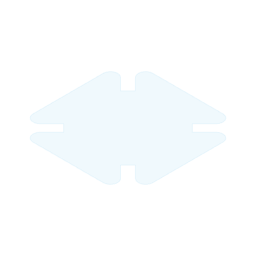
press-fit v4 (Autodesk Fusion 360 design; units mm, degrees)
Autodesk Fusion 360 part; units mm, degrees
sketch "Sketch1" plane through (0, 0, 0) normal (0, 0, 1) x (1, 0, 0)
sketch "Sketch2" plane through (0, 0, 0) normal (0, 0, 1) x (1, 0, 0)
  line L0 (-0.1061, 25.1061) -> (49.8939, 25.1061)
  line L1 (49.8939, 25.1061) -> (49.8939, -24.8939)
  line L2 (49.8939, -24.8939) -> (-0.1061, -24.8939)
  line L3 (-0.1061, -24.8939) -> (-0.1061, 25.1061)
  line L4 (9.8939, -14.8939) -> (9.8939, 15.1061)
  line L5 (9.8939, 15.1061) -> (39.8939, 15.1061)
  line L6 (39.8939, 15.1061) -> (39.8939, -14.8939)
  line L7 (39.8939, -14.8939) -> (9.8939, -14.8939)
  line L8 (-0.1061, -24.8939) -> (49.8939, 25.1061) construction
  line L9 (-0.1061, 25.1061) -> (49.8939, -24.8939) construction
  line L10 (-1.6263, -23.3737) -> (48.3737, 26.6264)
  line L11 (-1.6617, 23.5504) -> (48.3383, -26.4496)
  line L12 (1.4496, 26.6617) -> (51.4496, -23.3383)
  line L13 (1.4142, -26.4142) -> (51.4142, 23.5858)
  line L14 (12.9345, -14.8939) -> (9.8939, -11.8534)
  line L15 (36.7827, -14.8939) -> (39.8939, -11.7827)
  line L16 (9.8939, 11.9948) -> (13.0052, 15.1061)
  line L17 (36.8534, 15.1061) -> (39.8939, 12.0655)
  dimension "d10" = 50
  dimension "d11" = 50
  dimension "d12" = 10
  dimension "test" = 4.3
  dimension "test2" = 4.3
  constraint horizontal L0
  constraint vertical L1
  constraint horizontal L2
  constraint vertical L3
  constraint symmetric L9 L11.start L12.start
  constraint symmetric L9 L11.end L12.end
  constraint symmetric L8 L10.start L13.start
  constraint symmetric L8 L10.end L13.end
  constraint coincident L13 L14.start
  constraint coincident L7 L14.start
  constraint coincident L10 L14.end
  constraint coincident L4 L14.end
  constraint perpendicular L10 L14
  constraint coincident L7 L15.start
  constraint coincident L11 L15.start
  constraint coincident L6 L15.end
  constraint coincident L12 L15.end
  constraint perpendicular L12 L15
  constraint coincident L11 L16.start
  constraint coincident L4 L16.start
  constraint coincident L5 L16.end
  constraint coincident L12 L16.end
  constraint perpendicular L12 L16
  constraint coincident L5 L17.start
  constraint coincident L10 L17.start
  constraint coincident L6 L17.end
  constraint coincident L13 L17.end
  constraint perpendicular L13 L17
  measures "d10" distance of L0.start L0.end
  measures "d11" distance of L0.start L2.end
  measures "test" distance of L10 L13
extrude "Extrude3" add sketch "Sketch2" along normal blind 4.4 contours L0 L5 L10 L12 | L3 L4 L10 L11 | L5 L10 L12 | L10 L11 L12 L16 | L4 L10 L11 | L10 L12 L13 L17 | L10 L11 L12 L13 | L10 L11 L13 L14 | L1 L6 L12 L13 | L6 L12 L13 | L11 L12 L13 L15 | L2 L7 L11 L13 | L7 L11 L13 makes body 1
extrude "Extrude2" add sketch "Sketch2" along normal blind 4.4 separate body contours L0 L5 L10 L12 | L3 L4 L10 L11 | L5 L10 L12 | L10 L11 L12 L16 | L4 L10 L11 | L10 L12 L13 L17 | L10 L11 L12 L13 | L10 L11 L13 L14 | L1 L6 L12 L13 | L6 L12 L13 | L11 L12 L13 L15 | L2 L7 L11 L13 | L7 L11 L13 makes body 2
sketch "Sketch4" plane through (0, 0, 0) normal (0, 0, 1) x (1, 0, 0)
fillet "Fillet2" radius 3 8 edges at (49.8939, 22.0655, 2.2) (46.8534, 25.1061, 2.2) (3.0052, 25.1061, 2.2) (-0.1061, 21.9948, 2.2) (2.9345, -24.8939, 2.2) (46.7827, -24.8939, 2.2) (49.8939, -21.7827, 2.2) (-0.1061, -21.8534, 2.2) on bodies 2
sketch "Sketch5" plane through (0, 0, 4.4) normal (0, 0, 1) x (-1, 0, 0)
  arc A0 (0.1061, 14.6107) -> (-5.0153, 16.7321) centre (-2.8939, 14.6107) ccw
  line L0 (-5.0153, 16.7321) -> (-9.8939, 11.8534)
  line L1 (-9.8939, 11.8534) -> (-12.9345, 14.8939)
  line L2 (-12.9345, 14.8939) -> (-8.0558, 19.7726)
  arc A1 (-8.0558, 19.7726) -> (-10.1771, 24.8939) centre (-10.1771, 21.8939) ccw
  line L3 (-10.1771, 24.8939) -> (-39.54, 24.8939)
  arc A2 (-39.54, 24.8939) -> (-41.6613, 19.7726) centre (-39.54, 21.8939) ccw
  line L4 (-41.6613, 19.7726) -> (-36.7827, 14.8939)
  line L5 (-36.7827, 14.8939) -> (-39.8939, 11.7827)
  line L6 (-39.8939, 11.7827) -> (-44.7726, 16.6613)
  arc A3 (-44.7726, 16.6613) -> (-49.8939, 14.54) centre (-46.8939, 14.54) ccw
  line L7 (-49.8939, 14.54) -> (-49.8939, -14.8229)
  arc A4 (-49.8939, -14.8229) -> (-44.7726, -16.9442) centre (-46.8939, -14.8229) ccw
  line L8 (-44.7726, -16.9442) -> (-39.8939, -12.0655)
  line L9 (-39.8939, -12.0655) -> (-36.8534, -15.1061)
  line L10 (-36.8534, -15.1061) -> (-41.7321, -19.9847)
  arc A5 (-41.7321, -19.9847) -> (-39.6107, -25.1061) centre (-39.6107, -22.1061) ccw
  line L11 (-39.6107, -25.1061) -> (-10.2478, -25.1061)
  arc A6 (-10.2478, -25.1061) -> (-8.1265, -19.9847) centre (-10.2478, -22.1061) ccw
  line L12 (-8.1265, -19.9847) -> (-13.0052, -15.1061)
  line L13 (-13.0052, -15.1061) -> (-9.8939, -11.9948)
  line L14 (-9.8939, -11.9948) -> (-5.0153, -16.8735)
  arc A7 (-5.0153, -16.8735) -> (0.1061, -14.7522) centre (-2.8939, -14.7522) ccw
  line L15 (0.1061, -14.7522) -> (0.1061, 14.6107)
fillet "Fillet3" radius 3 8 edges at (46.7827, -24.8939, 2.2) (49.8939, -21.7827, 2.2) (2.9345, -24.8939, 2.2) (-0.1061, -21.8534, 2.2) (49.8939, 22.0655, 2.2) (46.8534, 25.1061, 2.2) (3.0052, 25.1061, 2.2) (-0.1061, 21.9948, 2.2) on bodies 1
sketch "Sketch6" plane through (0, 0, 4.4) normal (0, 0, 1) x (-1, 0, 0)
  arc A0 (-5.0153, -16.8735) -> (0.1061, -14.7522) centre (-2.8939, -14.7522) ccw
  line L0 (0.1061, -14.7522) -> (0.1061, 14.6107)
  arc A1 (0.1061, 14.6107) -> (-5.0153, 16.7321) centre (-2.8939, 14.6107) ccw
  line L1 (-5.0153, 16.7321) -> (-9.8939, 11.8534)
  line L2 (-9.8939, 11.8534) -> (-12.9345, 14.8939)
  line L3 (-12.9345, 14.8939) -> (-8.0558, 19.7726)
  arc A2 (-8.0558, 19.7726) -> (-10.1771, 24.8939) centre (-10.1771, 21.8939) ccw
  line L4 (-10.1771, 24.8939) -> (-39.54, 24.8939)
  arc A3 (-39.54, 24.8939) -> (-41.6613, 19.7726) centre (-39.54, 21.8939) ccw
  line L5 (-41.6613, 19.7726) -> (-36.7827, 14.8939)
  line L6 (-36.7827, 14.8939) -> (-39.8939, 11.7827)
  line L7 (-39.8939, 11.7827) -> (-44.7726, 16.6613)
  arc A4 (-44.7726, 16.6613) -> (-49.8939, 14.54) centre (-46.8939, 14.54) ccw
  line L8 (-49.8939, 14.54) -> (-49.8939, -14.8229)
  arc A5 (-49.8939, -14.8229) -> (-44.7726, -16.9442) centre (-46.8939, -14.8229) ccw
  line L9 (-44.7726, -16.9442) -> (-39.8939, -12.0655)
  line L10 (-39.8939, -12.0655) -> (-36.8534, -15.1061)
  line L11 (-36.8534, -15.1061) -> (-41.7321, -19.9847)
  arc A6 (-41.7321, -19.9847) -> (-39.6107, -25.1061) centre (-39.6107, -22.1061) ccw
  line L12 (-39.6107, -25.1061) -> (-10.2478, -25.1061)
  arc A7 (-10.2478, -25.1061) -> (-8.1265, -19.9847) centre (-10.2478, -22.1061) ccw
  line L13 (-8.1265, -19.9847) -> (-13.0052, -15.1061)
  line L14 (-13.0052, -15.1061) -> (-9.8939, -11.9948)
  line L15 (-9.8939, -11.9948) -> (-5.0153, -16.8735)
extrude "Extrude1" [suppressed]
fillet "Fillet1" [suppressed]
sketch "Sketch3" plane through (0, 0, 4.6) normal (0, 0, 1) x (-1, 0, 0)
  arc A0 (-50, -16.5567) -> (-46.3297, -18.077) centre (-47.85, -16.5567) ccw
  line L0 (-46.3297, -18.077) -> (-40, -11.7473)
  line L1 (-40, -11.7473) -> (-40, -15)
  line L2 (-40, -15) -> (-36.7473, -15)
  line L3 (-36.7473, -15) -> (-43.077, -21.3297)
  arc A1 (-43.077, -21.3297) -> (-41.5567, -25) centre (-41.5567, -22.85) ccw
  line L4 (-41.5567, -25) -> (-8.4433, -25)
  arc A2 (-8.4433, -25) -> (-6.923, -21.3297) centre (-8.4433, -22.85) ccw
  line L5 (-6.923, -21.3297) -> (-13.2527, -15)
  line L6 (-13.2527, -15) -> (-10, -15)
  line L7 (-10, -15) -> (-10, -11.7473)
  line L8 (-10, -11.7473) -> (-3.6703, -18.077)
  arc A3 (-3.6703, -18.077) -> (0, -16.5567) centre (-2.15, -16.5567) ccw
  line L9 (0, -16.5567) -> (0, 16.5567)
  arc A4 (0, 16.5567) -> (-3.6703, 18.077) centre (-2.15, 16.5567) ccw
  line L10 (-3.6703, 18.077) -> (-10, 11.7473)
  line L11 (-10, 11.7473) -> (-10, 15)
  line L12 (-10, 15) -> (-13.2527, 15)
  line L13 (-13.2527, 15) -> (-6.923, 21.3297)
  arc A5 (-6.923, 21.3297) -> (-8.4433, 25) centre (-8.4433, 22.85) ccw
  line L14 (-8.4433, 25) -> (-41.5567, 25)
  arc A6 (-41.5567, 25) -> (-43.077, 21.3297) centre (-41.5567, 22.85) ccw
  line L15 (-43.077, 21.3297) -> (-36.7473, 15)
  line L16 (-36.7473, 15) -> (-40, 15)
  line L17 (-40, 15) -> (-40, 11.7473)
  line L18 (-40, 11.7473) -> (-46.3297, 18.077)
  arc A7 (-46.3297, 18.077) -> (-50, 16.5567) centre (-47.85, 16.5567) ccw
  line L19 (-50, 16.5567) -> (-50, -16.5567)
hidden bodies 1 2
equation "edge_length = 50 mm"
equation "thickness = 4.4 mm"
equation "notch_length = 10 mm"
equation "kerf = 0.3 mm"
equation "d10 = edge_length"
equation "d11 = edge_length"
equation "d17 = thickness"
equation "d21 = thickness"
equation "test = 4.6 mm - kerf"
equation "test2 = 4.6 mm - kerf"
equation "d27 = thickness"
